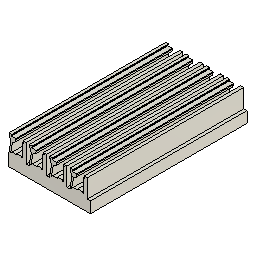
Parametric_Strip_Feeder (Autodesk Fusion 360 design; units mm, degrees)
Autodesk Fusion 360 part; units mm, degrees
note: some values were not read from the file. Set by a fixed rule: which sketch regions a step uses.
sketch "Skizze1" plane through (0, 0, 0) normal (0, 1, 0) x (1, 0, 0)
  line L0 (9.4, -17.7) -> (9.4, -18)
  line L1 (8.5, -17.7) -> (9.4, -17.7)
  line L2 (1.2293, -14.7) -> (0.1, -17.7)
  line L3 (4.3, -17.7) -> (4.3, -17.1)
  line L4 (0, -8.1) -> (1.2293, -14.7)
  line L5 (0.1, -18.9) -> (1.9, -18.9)
  line L6 (0.1, -17.7) -> (0.1, -18.9)
  line L7 (1.9, -18.4) -> (1.5, -18)
  line L8 (1.5, -18) -> (1.5, -17.7)
  line L9 (1.9, -18.9) -> (1.9, -18.4)
  line L10 (4.3, -17.1) -> (2.2465, -14.7)
  line L11 (13, 0) -> (0, 0)
  line L12 (9, -18.9) -> (11, -18.9)
  line L13 (0, 0) -> (0, -8.1)
  line L14 (8.5, -9.1) -> (8.5, -17.7)
  line L15 (4.3, -17.7) -> (1.5, -17.7)
  line L16 (11, -18.9) -> (11, -7.1)
  line L17 (9.4, -18) -> (9, -18.4)
  line L18 (9, -18.4) -> (9, -18.9)
  line L19 (4.9, -9.1) -> (2.0366, -9.1)
  line L20 (1.0172, -8.1) -> (2.2465, -14.7)
  line L21 (2.0366, -9.1) -> (1.0172, -8.1)
  line L22 (11, -7.1) -> (13, -7.1)
  line L23 (13, -7.1) -> (13, 0)
  circle A0 centre (12.5, -6.6) radius 0.5
  line L24 (2.2465, -14.7) -> (4, -15.7124)
  line L25 (2.2465, -14.7) -> (2.2465, -9.6844) construction
  line L26 (4.3, -17.1) -> (4, -15.7124)
  line L27 (0.7, -6.388) -> (0.7, -1)
  line L28 (0.7, -1) -> (12.5, -1)
  line L29 (12.5, -1) -> (12.5, -6.7)
  line L30 (12.5, -6.7) -> (10.6, -6.7)
  line L31 (10.6, -8.1) -> (10.6, -6.7)
  line L32 (4.9, -9.1) -> (4.9, -9.7)
  line L33 (4.9, -9.7) -> (7.9, -9.7)
  line L34 (7.9, -9.7) -> (7.9, -9.1)
  line L35 (7.9, -9.1) -> (8.5, -9.1)
  line L36 (8.5, -8.1) -> (10.6, -8.1)
  line L37 (1.7175, -7.3861) -> (0.7, -6.388)
  line L38 (6.9, -8.1) -> (8.5, -8.1)
  line L39 (6.9, -8.7) -> (6.9, -8.1)
  line L40 (5.9, -8.7) -> (6.9, -8.7)
  line L41 (5.9, -8.1) -> (5.9, -8.7)
  line L42 (5.9, -8.1) -> (2.4452, -8.1)
  line L43 (2.4452, -8.1) -> (1.7175, -7.3861)
  dimension "d14" = 7.9
  dimension "d15" = 2.8
  dimension "d16" = 0.9
  dimension "d17" = 17.7
  dimension "d18" = 0.3
  dimension "d21" = 18.9
  dimension "d26" = 35
  dimension "d28" = 1
  dimension "d30" = 150
  dimension "d31" = 0.4
  dimension "d32" = 1.4
  dimension "d33" = 1
  dimension "d34" = 0.6
  dimension "d35" = 3
  dimension "d36" = 45
  dimension "d37" = 45
  dimension "d38" = 0.4
  dimension "d39" = 0.1
  dimension "d42" = 1
  dimension "d94" = 2.5
  dimension "d95" = 0.5
  dimension "d96" = 0.5
  dimension "d97" = 2
  dimension "d98" = 1
  dimension "d105" = 120
  dimension "d106" = 2.5
  dimension "d119" = 8.6
  dimension "d135" = 1
  dimension "d136" = 0.7
  dimension "d137" = 0.5
  dimension "d139" = 0.4
  dimension "d141" = 0.4
  dimension "d142" = 0.6
  dimension "d143" = 0.6
  dimension "d144" = 8
  dimension "d146" = -1
  constraint perpendicular L3 L15
  constraint coincident L8.end L15.end
  constraint horizontal L1
  constraint coincident L0.start L1.end
  constraint horizontal L15
  constraint collinear L1 L15
  constraint coincident L2.end L6.start
  constraint coincident L2.start L4.end
  constraint coincident L5.end L9.start
  constraint perpendicular L15 L18
  constraint coincident L12.start L18.end
  constraint coincident L12.end L16.start
  constraint vertical L16
  constraint collinear L5 L12
  constraint coincident L7.start L9.end
  constraint vertical L9
  constraint coincident L3.end L10.start
  constraint vertical L8
  constraint vertical L6
  constraint vertical L13
  constraint perpendicular L14 L19
  constraint horizontal L19
  constraint coincident L20.start L21.end
  constraint parallel L4 L20
  constraint coincident L4.start L13.end
  constraint horizontal L4.start L20.start
  constraint coincident L11.end L13.start
  constraint horizontal L10.end L2.start
  constraint horizontal L2.end L8.end
  constraint horizontal L0.end L7.end
  constraint coincident L16 L22.start
  constraint perpendicular L22 L23
  constraint horizontal L22
  constraint coincident L16.end L22.start
  constraint coincident L11.start L23.end
  constraint vertical L25
  constraint coincident L24.end L26.end
  constraint vertical L27
  constraint perpendicular L27 L28
  constraint perpendicular L28 L29
  constraint perpendicular L29 L30
  constraint coincident L30.end L31.end
  constraint perpendicular L19 L32
  constraint perpendicular L32 L33
  constraint perpendicular L33 L34
  constraint perpendicular L34 L35
  constraint coincident L14.start L35.end
  constraint collinear L19 L35
  constraint coincident L31.start L36.end
  constraint coincident L27.start L37.end
  constraint parallel L37 L43
  measures "d14" distance of L0 L8
  measures "d15" distance of L3.start L8.end
  measures "d16" distance of L1.start L0.start
  measures "d17" distance of L11 L15
  measures "d18" distance of L8.end L7.end
  measures "d21" distance of L5 L11
  measures "d26" angle of L20 L21
  measures "d28" distance of L19 L20.start
  measures "d30" angle of L10 L20
  measures "d31" distance of L8 L9
  measures "d32" distance of L6 L8
  measures "d33" distance of L4 L20
  measures "d34" distance of L3.start L3.end
  measures "d35" distance of L10.end L15
  measures "d36" angle of L7 L8
  measures "d37" angle of L0 L17
  measures "d38" distance of L0 L18
  measures "d39" distance of L6 L13
  measures "d42" distance of L20.start L22
  measures "d94" distance of L14 L16
  measures "d95" distance of L23 A0.centre
  measures "d96" distance of L22 A0.centre
  measures "d97" distance of L16.end L22.end
  measures "d98" diameter of A0
  measures "d105" angle of L24 L25
  measures "d106" distance of L8 L24.end
  measures "d119" distance of L15 L19
  measures "d135" distance of L11 L28
  measures "d136" distance of L13 L27
  measures "d137" distance of L23 L29
  measures "d139" distance of L22 L30
  measures "d141" distance of L16 L31
  measures "d142" distance of L34.end L14.start
  measures "d143" distance of L3.start L32
  measures "d144" distance of L15 L33
extrude "Extrusion2" add sketch "Skizze1" along normal blind 1 contours A0 L29 L30 | A0 L29 L30
extrude "Extrusion1" add sketch "Skizze1" along normal blind 100
sketch "Skizze6" plane through (0, 0, 17.7) normal (0, 0, 1) x (-1, 0, 0)
  line L0 (-1.5, 0) -> (-4.3, 0)
  line L1 (-4.3, 0) -> (-4.3, -100)
  line L2 (-4.3, -100) -> (-1.5, -100)
  line L3 (-1.5, -100) -> (-1.5, 0)
  circle A0 centre (-3.25, -1.75) radius 0.75
  dimension "d99" = 1.5
  dimension "d100" = 1.75
  dimension "d102" = 1.75
  measures "d99" diameter of A0
  measures "d100" distance of L3 A0.centre
  measures "d102" distance of L0 A0.centre
sketch "Skizze4" plane through (0, 0, 0) normal (0, 0, -1) x (0, 1, 0)
  line L0 (0, 13) -> (0, 0)
  line L1 (100, 0) -> (100, 13)
  line L2 (0, 0) -> (0, 13)
  line L3 (0, 0) -> (-10, 0)
  line L4 (-10, 0) -> (-10, 13)
  line L5 (-10, 13) -> (0, 13)
  line L6 (50, 0) -> (50, 17.319) construction
  circle A0 centre (-5, 6.5) radius 1.65
  line L7 (100, 0) -> (110, 0)
  line L8 (100, 0) -> (100, 13)
  line L9 (110, 13) -> (100, 13)
  line L10 (110, 0) -> (110, 13)
  circle A1 centre (105, 6.5) radius 1.65
  line L11 (0, 0) -> (100, 0)
  line L12 (100, 13) -> (0, 13)
  circle A2 centre (105, 6.5) radius 4
  circle A3 centre (-5, 6.5) radius 4
  point P0 (-10, 6.5)
  point P1 (-5, 0)
  point P2 (0, 13)
  dimension "d88" = 3.3
  dimension "d89" = 10
  dimension "d123" = 8
  constraint perpendicular L2 L3
  constraint perpendicular L3 L4
  constraint perpendicular L4 L5
  constraint coincident P2 L0.start
  constraint midpoint L4 P0
  constraint midpoint L3 P1
  constraint horizontal A0.centre P0
  constraint vertical A0.centre P1
  constraint symmetric L0.end L6 L1.start
  constraint symmetric P2 L6 L1.end
  constraint symmetric L3.end L6 L7.end
  constraint symmetric L4.end L6 L9.start
  constraint symmetric L6 A0 A1
  constraint midpoint L6.start L11
  constraint coincident L1.start L7.start
  constraint horizontal L3
  constraint vertical L6
  constraint coincident P2 L5
  constraint concentric A1 A2
  constraint concentric A0 A3
  constraint equal A2 A3
  measures "d88" diameter of A0
  measures "d89" distance of L0.end L3.end
  measures "d123" diameter of A3
pattern_linear "R-Anordnung1" count 4 spacing 13 along (-1, 0, 0) of "Extrusion1"
equation "Strip_width = 8 mm" comment "check!!! 8, 12, 16, 24 mm"
equation "Strip_hight = 0.3 mm" comment "check!!! default: 0,7; paper strip 0,9mm; plastic strip 0,3mm"
equation "Reference_hight_machine = 18 mm" comment "Pickuphight from table"
equation "Number_Feeders = 4" comment "check!!! Amount of Strips"
equation "Length_Strips = 100 mm" comment "check!!! Strip Length"
equation "Tape_Clearence = 0.1 mm" comment "default 0,05"
equation "TapeSupport_width_HoleSide = 2.8 mm"
equation "TapeSupport_width_NonHoleSide = 0.9 mm"
equation "With_between_feeders = 2 mm"
equation "d14 = Strip_width - Tape_Clearence"
equation "d15 = TapeSupport_width_HoleSide"
equation "d16 = TapeSupport_width_NonHoleSide"
equation "d17 = Reference_hight_machine - Strip_hight"
equation "d18 = Strip_hight"
equation "d21 = Reference_hight_machine + 0.9 mm"
equation "d37 = d36"
equation "d38 = d31"
equation "d39 = Tape_Clearence"
equation "d40 = Length_Strips"
equation "d44 = Number_Feeders"
equation "d46 = -3 mm - Strip_width - With_between_feeders"
equation "width = 3 mm"
equation "d95 = d98 / 2"
equation "d96 = d98 / 2"
equation "d97 = With_between_feeders"
equation "Strip_Pitch = 4 mm"
equation "d102 = d100"
equation "d105 = 30 deg + 90 deg"
equation "Components_max_height = 8 mm" comment "default 8mm"
equation "d141 = d139"
equation "d142 = d143"
equation "d144 = Components_max_height"
named bodies: "Strip_Feeder"
